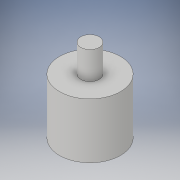
# Autodesk Inventor part: Motor
Saved by Autodesk Inventor 2019 (Build 230136000, 136)
## iProperties
Created: 2019-06-19
Part Number: Motor
Material: Generic
Document SubType Name: Modeling
Designer: abdel
Density: 1 g/cm^3
Appearance: Default
Author: abdel
Autodesk Inventor part; units mm, degrees
ref_plane "YZ Plane" through (0, 0, 0) normal (1, 0, 0) x (0, 1, 0)
ref_plane "XZ Plane" through (0, 0, 0) normal (0, 1, 0) x (-1, 0, 0)
ref_plane "XY Plane" through (0, 0, 0) normal (0, 0, 1) x (1, 0, 0)
sketch "Sketch1" plane through (0, 0, 0) normal (0, 1, 0) x (-1, 0, 0)
  circle A0 centre (0, 0) radius 4.2386
  circle A1 centre (0, 0) radius 14.0056
  dimension "d0" = 8.4772
  dimension "d1" = 28.0111
  constraints: 2 centre point, 2 coincident
  measures "d0" diameter of A0
  measures "d1" diameter of A1
extrude "Extrusion1" add sketch "Sketch1" along normal blind 25.4 contours A0 | A1
sketch "Sketch2" plane through (0, 25.4, 0) normal (0, 1, 0) x (1, 0, 0)
  circle A0 centre (0, 0) radius 4.2386
  circle A1 centre (0, 0) radius 14.0056
  dimension "d4" = 8.4772
  dimension "d5" = 28.0111
  constraints: 2 centre point, 2 coincident
  measures "d4" diameter of A0
  measures "d5" diameter of A1
extrude "Extrusion2" add sketch "Sketch2" along normal blind 12.7 contours A0
body "Solid1"
